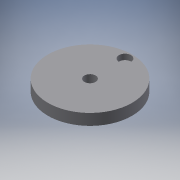
# Autodesk Inventor part: sensor wheel
Saved by Autodesk Inventor 2016 (Build 200138000, 138)
## iProperties
Created: 2017-06-15
Part Number: sensor wheel
Material: Generic
Document SubType Name: Modeling
Designer: RMcComber
Density: 1 g/cm^3
Appearance: Default
Author: RMcComber
Autodesk Inventor part; units mm, degrees
ref_plane "YZ Plane" through (0, 0, 0) normal (1, 0, 0) x (0, 1, 0)
ref_plane "XZ Plane" through (0, 0, 0) normal (0, 1, 0) x (-1, 0, 0)
ref_plane "XY Plane" through (0, 0, 0) normal (0, 0, 1) x (1, 0, 0)
sketch "Sketch1" plane through (0, 0, 0) normal (0, 0, 1) x (1, 0, 0)
  circle A0 centre (0, 0) radius 30
  circle A1 centre (0, 0) radius 4
  dimension "d0" = 60
  dimension "d1" = 8
  constraints: 2 centre point, 2 coincident
  measures "d0" diameter of A0
  measures "d1" diameter of A1
extrude "Extrusion1" add sketch "Sketch1" along normal blind 8
sketch "Sketch2" plane through (0, 0, 8) normal (0, 0, 1) x (1, 0, 0)
  circle A0 centre (0, 0) radius 30 projected
  line L0 (0, 0) -> (0, 25) construction
  circle A1 centre (0, 25) radius 4.25
  dimension "d4" = 8.5
  dimension "d5" = 25
  constraints: 2 end point, 1 centre point, 1 coincident, 1 vertical
  measures "d4" diameter of A1
  measures "d5" distance of L0.start L0.end
extrude "Extrusion2" cut sketch "Sketch2" against normal blind 4 contours A1
sketch "Sketch3" plane through (0, 0, 0) normal (0, 0, -1) x (-1, 0, 0)
  circle A0 centre (0, 0) radius 4 projected
  line L0 (-4, 0) -> (-12.5, 0)
  line L1 (-12.5, 0) -> (-12.5, -10)
  line L2 (-12.5, -10) -> (12.5, -10)
  line L3 (12.5, -10) -> (12.5, 0)
  line L4 (12.5, 0) -> (4, 0)
  dimension "d8" = 10
  dimension "d9" = 25
  constraints: 10 end point, 3 collinear, 2 parallel, 2 point on circle, 1 horizontal, 1 horizontal alignment, 1 perpendicular
  measures "d8" distance of L0.end L1.end
  measures "d9" distance of L1.end L2.end
extrude "Extrusion3" add sketch "Sketch3" along normal blind 6 contours L4 L3 L2 L1 L0 A0
sketch "Sketch4" plane through (4, 0, 0) normal (0, 1, 0) x (1, 0, 0)
  line L0 (8.5, 0) -> (0, 0) projected
  line L1 (0, 6) -> (8.5, 6) projected
  line L2 (-8, 0) -> (-16.5, 0) projected
  line L3 (-8, 0) -> (-8, 6) projected
  line L4 (-16.5, 6) -> (-8, 6) projected
  line L5 (-16.5, 0) -> (-16.5, 6) projected
  line L6 (-12.25, 6) -> (-12.25, 0) construction
  line L7 (4.25, 6) -> (4.25, 0) construction
  circle A0 centre (-12.25, 3) radius 1.4
  circle A1 centre (4.25, 3) radius 1.4
  point P0 (-4, 0)
  dimension "d12" = 2.8
  constraints: 6 midpoint, 4 end point, 2 centre point, 1 equal radius
  measures "d12" diameter of A0
extrude "Extrusion4" cut sketch "Sketch4" against normal through all contours A0 | A1
body "Solid1"
